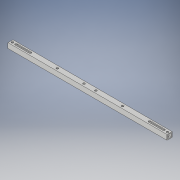
# Autodesk Inventor part: holder_bar
Saved by Autodesk Inventor 2019 (Build 230136000, 136)
## iProperties
Created: 2019-02-02
Part Number: holder_bar
Material: Generic
Document SubType Name: Modeling
Designer: suchanek
Density: 1 g/cm^3
Appearance: Default
Author: suchanek
Autodesk Inventor part; units mm, degrees
ref_plane "YZ Plane" through (0, 0, 0) normal (1, 0, 0) x (0, 1, 0)
ref_plane "XZ Plane" through (0, 0, 0) normal (0, 1, 0) x (-1, 0, 0)
ref_plane "XY Plane" through (0, 0, 0) normal (0, 0, 1) x (1, 0, 0)
sketch "Sketch1" plane through (0, 0, 0) normal (1, 0, 0) x (0, 1, 0)
  line L0 (-6.35, 6.35) -> (6.35, 6.35)
  line L1 (6.35, 6.35) -> (6.35, -6.35)
  line L2 (6.35, -6.35) -> (-6.35, -6.35)
  line L3 (-6.35, -6.35) -> (-6.35, 6.35)
  line L4 (-6.35, 6.35) -> (6.35, -6.35) construction
  line L5 (6.35, 6.35) -> (-6.35, -6.35) construction
  line L6 (-4.35, 4.35) -> (4.35, 4.35)
  line L7 (4.35, 4.35) -> (4.35, -4.35)
  line L8 (4.35, -4.35) -> (-4.35, -4.35)
  line L9 (-4.35, -4.35) -> (-4.35, 4.35)
  line L10 (-4.35, 4.35) -> (4.35, -4.35) construction
  line L11 (4.35, 4.35) -> (-4.35, -4.35) construction
  point P0 (0, 0)
  dimension "d0" = 12.7
  dimension "d1" = 12.7
  dimension "d15" = 2
  dimension "d16" = 2
  constraints: 24 end point, 4 midpoint, 4 parallel, 2 horizontal, 2 perpendicular
  measures "d0" distance of L1.end L2.end
  measures "d1" distance of L0.end L1.end
  measures "d15" distance between parallel lines of L1 L7
  measures "d16" distance between parallel lines of L2 L8
extrude "Extrusion1" add sketch "Sketch1" along normal mid plane 400
sketch "Sketch2" plane through (-200, 6.35, 6.35) normal (0, 1, 0) x (1, 0, 0)
  circle A0 centre (5, 6.35) radius 2.6
  line L0 (14, 6.35) -> (50, 6.35) construction
  line L1 (14, 3.75) -> (50, 3.75)
  line L2 (50, 8.95) -> (14, 8.95)
  arc A1 (14, 8.95) -> (14, 3.75) centre (14, 6.35) ccw
  arc A2 (50, 3.75) -> (50, 8.95) centre (50, 6.35) ccw
  line L3 (0, 0) -> (0, 12.7) projected
  circle A3 centre (118, 6.35) radius 2.6
  circle A4 centre (185, 6.35) radius 2.6
  point P0 (200, 6.35)
  point P1 (32, 6.35)
  dimension "d6" = 5.2
  dimension "d7" = 5
  dimension "d8" = 9
  dimension "d9" = 36
  dimension "d13" = 67
  dimension "d14" = 15
  constraints: 8 end point, 5 centre point, 4 point on circle, 4 point on line, 4 tangent, 3 equal radius, 1 horizontal, 1 midpoint, 1 parallel
  measures "d6" diameter of A0
  measures "d7" distance from line of L3 A0.centre
  measures "d8" distance of A0.centre L0.start
  measures "d9" distance of L2.start L2.end
  measures "d13" distance of A3.centre A4.centre
  measures "d14" distance of point (200, 6.35) A4.centre
extrude "Extrusion2" cut sketch "Sketch2" against normal blind 100
mirror "Mirror1" about plane through (0, 0, 0) normal (1, 0, 0) of "Extrusion2"
body "Solid1"
